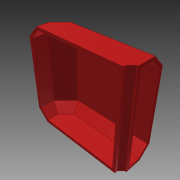
# Autodesk Inventor part: power_supply_fan_chamber
Saved by Autodesk Inventor 2014 (Build 180170000, 170)
## iProperties
Created: 2013-12-19
Part Number: power_supply_fan_chamber
Material: ABS Plastic
Document SubType Name: Modeling
Designer: buben
Density: 1.06 g/cm^3
Appearance: Light Red
Author: buben
Autodesk Inventor part; units mm, degrees
ref_plane "YZ Plane" through (0, 0, 0) normal (1, 0, 0) x (0, 1, 0)
ref_plane "XZ Plane" through (0, 0, 0) normal (0, 1, 0) x (-1, 0, 0)
ref_plane "XY Plane" through (0, 0, 0) normal (0, 0, 1) x (1, 0, 0)
sketch "Sketch1" plane through (0, 0, 0) normal (0, 0, 1) x (1, 0, 0)
  line L0 (0, 0) -> (0, 12)
  line L1 (0, 12) -> (13, 25)
  line L2 (13, 25) -> (72, 25)
  line L3 (68, 0) -> (68, 2)
  line L4 (68, 2) -> (71, 5)
  line L5 (71, 5) -> (72, 5)
  line L6 (72, 5) -> (72, 25)
  line L7 (68, 0) -> (0, 0)
  point P0 (34, 0)
  dimension "d1" = 45
  dimension "d2" = 25
  dimension "d3" = 68
  dimension "d4" = 5
  dimension "d5" = 2
  dimension "d6" = 12
  dimension "d7" = 38
  constraints: 16 end point, 4 perpendicular, 2 parallel, 1 midpoint, 1 vertical
  measures "d1" angle of L0 L1
  measures "d2" vertical distance of L3.start L2.end
  measures "d3" distance of L3.start L0.start
  measures "d4" distance from line of L3.start L5
  measures "d5" distance of L3.start L3.end
  measures "d6" distance of L0.start L0.end
  measures "d7" distance from line of point (34, 0) L6
extrude "Extrusion1" add sketch "Sketch1" along normal blind 68
chamfer "Chamfer1" distance 8 angle 45 6 edges at (0, 6, 68) (6.5, 18.5, 68) (42.5, 25, 68) (0, 6, 0) (6.5, 18.5, 0) (42.5, 25, 0)
shell "Shell1" thickness 2 removed faces 2 at (48, 0, 45.3333) at (72, 11.6667, 25.3333)
body "Solid1"
